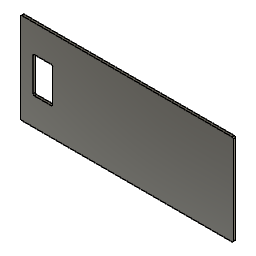
lid (Autodesk Fusion 360 design; units mm, degrees)
Autodesk Fusion 360 part; units mm, degrees
sketch "Sketch1" plane through (0, 0, 0) normal (0, 1, 0) x (1, 0, 0)
  line L0 (0, 0) -> (185, 0)
  line L1 (185, 0) -> (185, -79)
  line L2 (185, -79) -> (0, -79)
  line L3 (0, -79) -> (0, 0)
  constraint horizontal L0
  constraint vertical L1
  constraint horizontal L2
  constraint vertical L3
  constraint coincident L0.start L3.end
extrude "Extrude1" add sketch "Sketch1" along normal blind 2
sketch "Sketch2" plane through (0, 0, 0) normal (0, 1, 0) x (1, 0, 0)
  line L0 (11, -24) -> (28, -24)
  line L1 (28, -24) -> (28, -55)
  line L2 (28, -55) -> (11, -55)
  line L3 (11, -55) -> (11, -24)
  constraint horizontal L0
  constraint vertical L1
  constraint horizontal L2
  constraint vertical L3
extrude "Extrude2" cut sketch "Sketch2" along normal blind 5
fillet "Fillet1" radius 1 1 edges at (185, 1, 79)
fillet "Fillet2" radius 1 1 edges at (185, 1, 0)
fillet "Fillet3" radius 1 1 edges at (0, 1, 79)
fillet "Fillet4" radius 1 1 edges at (0, 1, 0)
fillet "Fillet5" radius 1 1 edges at (28, 1, 55)
fillet "Fillet6" radius 1 1 edges at (11, 1, 55)
fillet "Fillet7" radius 1 1 edges at (11, 1, 24)
fillet "Fillet8" radius 1 1 edges at (28, 1, 24)
